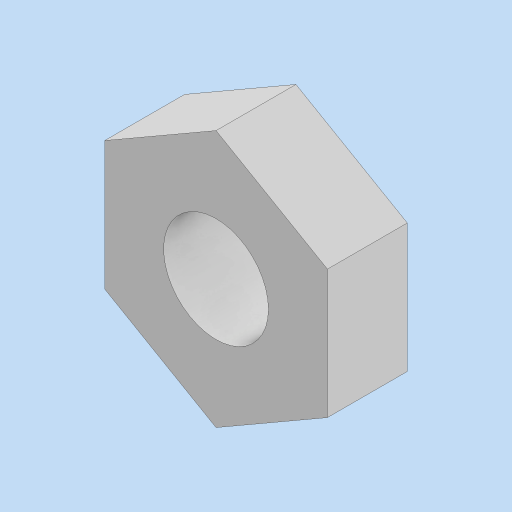
# Autodesk Inventor part: tuerca2mockup
Saved by Autodesk Inventor 2024 (Build 280153000, 153)
## iProperties
Created: 2024-09-12
Part Number: tuerca2mockup
Material: Generic
Document SubType Name: Modeling
Designer: MxMon
Density: 1 g/cm^3
Appearance: Default
Author: MxMon
Autodesk Inventor part; units mm, degrees
ref_plane "YZ Plane" through (0, 0, 0) normal (1, 0, 0) x (0, 1, 0)
ref_plane "XZ Plane" through (0, 0, 0) normal (0, 1, 0) x (-1, 0, 0)
ref_plane "XY Plane" through (0, 0, 0) normal (0, 0, 1) x (1, 0, 0)
sketch "Sketch1" plane through (0, 0, 0) normal (0, 0, 1) x (1, 0, 0)
  circle A0 centre (0, 0) radius 2
  arc A1 (-1.8366, -0.7917) -> (1.544, 1.2713) centre (0, 0) ccw
  arc A2 (1.544, 1.2713) -> (-1.8366, -0.7917) centre (0, 0) ccw
  line L0 (0, -4.9075) -> (-4.25, -2.4537)
  line L1 (-4.25, -2.4537) -> (-4.25, 2.4537)
  line L2 (-4.25, 2.4537) -> (0, 4.9075)
  line L3 (0, 4.9075) -> (4.25, 2.4537)
  line L4 (4.25, 2.4537) -> (4.25, -2.4537)
  line L5 (4.25, -2.4537) -> (0, -4.9075)
  point P0 (-2.125, 3.6806)
  point P1 (4.25, 0)
  dimension "d8" = 8.5
  dimension "d9" = 4
  constraints: 12 end point, 6 point on circle, 3 centre point, 3 coincident, 2 concentric, 2 midpoint, 1 horizontal alignment, 1 vertical alignment, 13 other
  measures "d8" distance from line of L5 point (-2.125, 3.681)
  measures "d9" diameter of A0
extrude "Extrusion2" add sketch "Sketch1" along normal blind 3.05
body "Solid2"
